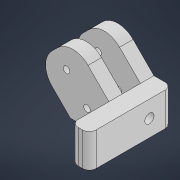
# Autodesk Inventor part: Idle belt holder
Saved by Autodesk Inventor 2022 (Build 260153000, 153)
## iProperties
Created: 2021-10-05
Part Number: Idle belt holder
Material: Generic
Document SubType Name: Modeling
Designer: Administrator
Density: 1 g/cm^3
Appearance: Default
Mass: 4.75917 g
Surface Area: 26.3693 cm^2
Volume: 4.75917 cm^3
Title: Idle belt holder v4
Author: Administrator
Autodesk Inventor part; units mm, degrees
ref_plane "YZ Plane" through (0, 0, 0) normal (1, 0, 0) x (0, 1, 0)
ref_plane "XY Plane" through (0, 0, 0) normal (0, 0, 1) x (1, 0, 0)
ref_plane "Work Plane1" through (0, -6.5, 0) normal (0, 1, 0) x (-1, 0, 0)
sketch "Sketch1" plane through (0, -6.5, 0) normal (0, 1, 0) x (-1, 0, 0)
  arc A0 (-2.625, 0) -> (0, -2.625) centre (0, 0) ccw
  line L0 (-2.625, 0) -> (-2.625, 26.85)
  arc A1 (0, 29.475) -> (-2.625, 26.85) centre (0, 26.85) ccw
  line L1 (4.375, 26.85) -> (4.375, 14.875)
  line L2 (16.75, 9.625) -> (4.375, 9.625)
  line L3 (0, 29.475) -> (1.75, 29.475)
  line L4 (4.375, 9.625) -> (4.375, 2.625)
  arc A2 (4.375, 26.85) -> (1.75, 29.475) centre (1.75, 26.85) ccw
  line L5 (4.375, 14.875) -> (16.75, 14.875)
  line L6 (16.75, -2.625) -> (0, -2.625)
  arc A3 (16.75, 9.625) -> (16.75, 14.875) centre (16.75, 12.25) ccw
  line L7 (4.375, 2.625) -> (16.75, 2.625)
  arc A4 (16.75, -2.625) -> (16.75, 2.625) centre (16.75, 0) ccw
  dimension "d35" = 7
  dimension "d36" = 7
  dimension "d37" = 12.375
  dimension "d38" = 5.25
  dimension "d39" = 14.6
  constraints: 16 end point, 10 point on circle, 9 tangent, 5 centre point, 5 horizontal, 4 equal radius, 3 vertical, 2 parallel, 1 coincident, 1 collinear
  measures "d35" distance of L2.end L4.end
  measures "d36" distance between parallel lines of L0 L1
  measures "d37" distance from line of L1 A3.centre
  measures "d38" distance between parallel lines of L2 L5
  measures "d39" distance between parallel lines of L3 L5
extrude "Extrusion2" add sketch "Sketch1" along normal blind 13
hole "Hole3" at (-12.875, 0, 9.625) direction (0, 0, 1) diameter 2.529 depth 5.25 tip angle 118
sketch "Sketch3" plane through (-4.375, -6.5, 9.625) normal (0, 0, -1) x (-1, 0, 0)
  point P0 (8.5, 6.5)
hole "Hole1" at (-12.875, 0, -2.625) direction (0, 0, 1) diameter 2.529 depth 5.25 tip angle 118
sketch "Sketch6" plane through (-16.75, -6.5, 14.875) normal (0, 0, 1) x (1, 0, 0)
  circle A0 centre (-4.0623, 15.5) radius 4.5
  circle A1 centre (3.875, 6.5) radius 4.5
  circle A2 centre (3.875, 6.5) radius 1.2645 projected
  line L0 (0, 0) -> (12.375, 0) projected
  line L1 (12.375, 0) -> (12.375, 13) projected
  line L2 (0, 13) -> (12.375, 13) projected
  line L3 (0, 0) -> (0, 13) projected
  circle A3 centre (3.875, 6.5) radius 1.2645 projected
  circle A4 centre (-4.0623, 15.5) radius 6.5
  circle A5 centre (3.875, 6.5) radius 6.5
  line L4 (3.875, 11) -> (-4.0623, 11)
  line L5 (0, 0) -> (0, 0) projected
  line L6 (0, 0) -> (0, 13) projected
  line L7 (0, 13) -> (0, 13) projected
  line L8 (0, 0) -> (0, 13) projected
  line L9 (-2.625, 0) -> (-2.625, 13) projected
  line L10 (-2.625, 0) -> (-15.6685, 13.1351)
  line L11 (-15.6685, 13.1351) -> (-1.6162, 27.0894)
  line L12 (12.375, 0) -> (12.375, 13) projected
  line L13 (-1.6162, 27.0894) -> (12.375, 13)
  line L14 (2.9639, 22.4772) -> (-11.0884, 8.5228)
  circle A6 centre (-4.0623, 15.5) radius 1.2645
  point P0 (16.75, 6.5)
  point P1 (-2.625, 11)
  point P2 (-0.8154, 11)
  point P3 (0, 11.7187)
  dimension "d26" = 9
  dimension "d27" = 9
  dimension "d28" = 2
  dimension "d29" = 2
  dimension "d30" = 1
  constraints: 10 end point, 3 centre point, 3 horizontal, 2 coincident, 2 perpendicular, 2 point on line, 2 vertical alignment, 1 equal radius, 1 midpoint, 1 parallel, 1 tangent, 6 other
extrude "Extrusion4" add sketch "Sketch6" against normal up to surface (5.25 mm away) contours A0 L14 A6 | A0 L14 A4 L2 L3 A5 L4 L9 | L14 A6 A0 | A0 L14 A4 | L9 L4 A0 | A0 L4 L9 A4 L14 | L14 L13 L2 A4 | A4 L11 L13 L14 | L14 L10 L11 A4 | A4 L9 L10 L14
sketch "Sketch7" plane through (0, -6.5, 0) normal (0, -1, 0) x (1, 0, 0)
  arc A0 (0, -2.625) -> (2.625, 0) centre (0, 0) ccw projected
  line L0 (2.625, 26.85) -> (2.625, 0) projected
  arc A1 (2.625, 26.85) -> (0, 29.475) centre (0, 26.85) ccw projected
  line L1 (-1.75, 29.475) -> (0, 29.475) projected
  arc A2 (-1.75, 29.475) -> (-4.375, 26.85) centre (-1.75, 26.85) ccw projected
  line L2 (-4.375, 14.875) -> (-4.375, 26.85) projected
  line L3 (-16.75, 14.875) -> (-4.375, 14.875) projected
  arc A3 (-16.75, 14.875) -> (-19.375, 12.25) centre (-16.75, 12.25) ccw projected
  arc A4 (-19.375, 12.25) -> (-16.75, 9.625) centre (-16.75, 12.25) ccw projected
  line L4 (-4.375, 9.625) -> (-16.75, 9.625) projected
  line L5 (-4.375, 2.625) -> (-4.375, 9.625) projected
  line L6 (-16.75, 2.625) -> (-4.375, 2.625) projected
  arc A5 (-16.75, 2.625) -> (-16.75, -2.625) centre (-16.75, 0) ccw projected
  line L7 (0, -2.625) -> (-16.75, -2.625) projected
  arc A6 (-17.5654, 14.7451) -> (-19.375, 12.25) centre (-16.75, 12.25) ccw projected
  line L8 (-17.5654, 14.875) -> (-17.5654, 14.7451) projected
  line L9 (-19.375, 14.875) -> (-17.5654, 14.875) projected
  line L10 (-19.375, 14.875) -> (-19.375, 12.25) projected
  line L11 (-32.4185, 9.625) -> (-19.375, 9.625) projected
  line L12 (-19.375, 12.25) -> (-19.375, 9.625) projected
  line L13 (-19.375, 14.875) -> (-19.375, 12.25) projected
  line L14 (-32.4185, 14.875) -> (-19.375, 14.875) projected
  line L15 (-32.4185, 14.875) -> (-32.4185, 9.625) projected
  arc A7 (-19.375, 12.25) -> (-17.5654, 9.7549) centre (-16.75, 12.25) ccw projected
  line L16 (-19.375, 12.25) -> (-19.375, 9.625) projected
  line L17 (-19.375, 9.625) -> (-17.5654, 9.625) projected
  line L18 (-17.5654, 9.7549) -> (-17.5654, 9.625) projected
  line L19 (-17.5654, 9.7549) -> (-17.5654, 9.625) projected
  line L20 (-17.5654, 9.625) -> (-16.75, 9.625) projected
  line L21 (-17.5654, 14.875) -> (-16.75, 14.875) projected
  line L22 (-17.5654, 14.875) -> (-17.5654, 14.7451) projected
  point P0 (-16.75, 9.625)
  constraints: 2 other
extrude "Extrusion5" add sketch "Sketch7" against normal blind 15 contours L20 L18 A4 | L18 L17 L12 A4 | A3 L8 L21 | L10 L9 L8 A3
ref_plane "Work Plane2" through (-4.375, -6.5, 6.125) normal (0, 0, -1) x (-1, 0, 0)
mirror "Mirror1" about plane through (-4.375, -6.5, 6.125) normal (0, 0, -1) of "Extrusion4", "Extrusion5"
fillet "Fillet1" radius 8.35 4 edges at (-32.4185, 6.6351, 12.25) (-18.3662, 20.5894, 12.25) (-18.3662, 20.5894, 0) (-32.4185, 6.6351, 0)
sketch "Sketch8" plane through (-4.375, -6.5, 2.625) normal (-1, 0, 0) x (0, 0, 1)
  line L0 (0, 0) -> (7, 0) projected
  line L1 (7, 0) -> (7, 13) projected
  line L2 (0, 13) -> (7, 13) projected
  line L3 (0, 0) -> (0, 13) projected
  line L4 (0, 0) -> (0, 13) projected
  line L5 (0, 6.5) -> (7, 6.5)
  line L6 (7, 0) -> (7, 13) projected
  point P0 (-2.625, 6.5)
  point P1 (3.5, 6.5)
  constraints: 3 midpoint, 2 end point
hole "Hole5" at (-4.375, 0, 6.125) direction (1, 0, 0) diameter 3.6 end through all counterbore diameter 6.5 counterbore depth 3 clearance for "Socket Head Cap Screw" size "M3" standard "Ansi Metric M Profile"
sketch "Sketch5" plane through (0, -6.5, -2.625) normal (0, 0, -1) x (-1, 0, 0)
  point P0 (12.875, 6.5)
body "Solid3"
